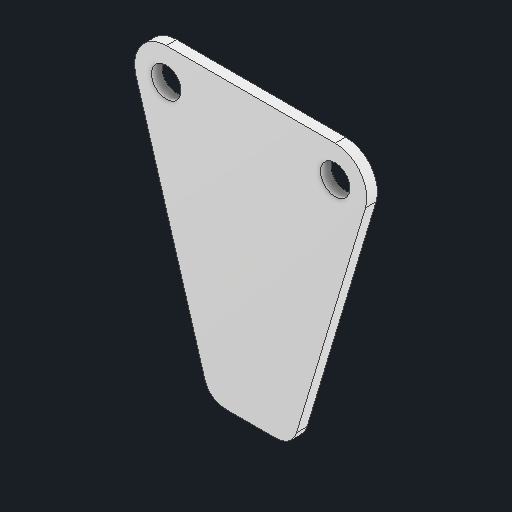
# Autodesk Inventor part: hoook_gusset
Saved by Autodesk Inventor 2025 (Build 290162000, 162)
## iProperties
Created: 2024-10-13
Part Number: hoook_gusset
Material: Acetal Resin, White
Document SubType Name: Modeling
Designer: Averey Ku
Density: 1.425 g/cm^3
Appearance: Smooth - White
Author: Averey Ku
Autodesk Inventor part; units mm, degrees
ref_plane "YZ Plane" through (0, 0, 0) normal (1, 0, 0) x (0, 1, 0)
ref_plane "XZ Plane" through (0, 0, 0) normal (0, 1, 0) x (-1, 0, 0)
ref_plane "XY Plane" through (0, 0, 0) normal (0, 0, 1) x (1, 0, 0)
sketch "Sketch1" plane through (0, 0, 0) normal (0, 0, 1) x (1, 0, 0)
  circle A0 centre (13.2036, 20.3187) radius 2.2225
  circle A1 centre (-12.1964, 20.3187) radius 2.2225
  arc A2 (17.764, 18.9458) -> (13.2036, 25.0812) centre (13.2036, 20.3187) ccw
  arc A3 (-12.1964, 25.0812) -> (-16.7567, 18.9458) centre (-12.1964, 20.3187) ccw
  line L0 (13.2036, 25.0812) -> (-12.1964, 25.0812)
  line L1 (7.3873, -15.5216) -> (17.764, 18.9458)
  line L2 (4.3471, -17.7813) -> (-3.3398, -17.7813)
  line L3 (-6.38, -15.5216) -> (-16.7567, 18.9458)
  arc A4 (4.3471, -17.7813) -> (7.3873, -15.5216) centre (4.3471, -14.6063) ccw
  arc A5 (-6.38, -15.5216) -> (-3.3398, -17.7813) centre (-3.3398, -14.6063) ccw
  point P0 (0, 0)
  point P1 (6.707, -17.7813)
  dimension "d0" = 38.1
  dimension "d1" = 3.175
  dimension "d2" = 4.7625
  dimension "d3" = 4.7625
  constraints: 8 end point, 8 point on circle, 7 tangent, 6 centre point, 2 coincident, 2 point on line, 1 equal radius, 1 horizontal
  measures "d0" vertical distance of A2.centre point (6.707, -17.781)
  measures "d1" radius of A4
  measures "d2" radius of A2
  measures "d3" radius of A3
extrude "Extrusion1" add sketch "Sketch1" along normal blind 1.5875
body "Solid1"
